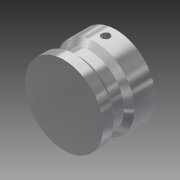
# Autodesk Inventor part: wheel_hub
Saved by Autodesk Inventor 2013 (Build 170138000, 138)
## iProperties
Created: 2013-07-22
Part Number: wheel_hub
Material: Generic
Document SubType Name: Modeling
Designer: dkboone
Density: 1 g/cm^3
Author: dkboone
Autodesk Inventor part; units mm, degrees
note: some values were not read from the file. Chosen so that the rebuilt part matches the saved one: direction of "Hole2".
ref_plane "YZ Plane" through (0, 0, 0) normal (1, 0, 0) x (0, 1, 0)
ref_plane "XY Plane" through (0, 0, 0) normal (0, 0, 1) x (1, 0, 0)
sketch "Sketch1" plane through (0, 0, 0) normal (1, 0, 0) x (0, 1, 0)
  line L0 (0, 0) -> (9.525, 0)
  line L1 (9.525, 0) -> (9.525, -2.54)
  line L2 (9.525, -2.54) -> (8.255, -3.81)
  line L3 (8.255, -3.81) -> (8.255, -6.35)
  line L4 (8.255, -6.35) -> (9.525, -7.62)
  line L5 (9.525, -7.62) -> (9.525, -12.7)
  line L6 (9.525, -12.7) -> (0, -12.7)
  line L7 (0, -12.7) -> (0, 0)
  line L8 (0, -15.24) -> (0, 2.54) projected
  dimension "d0" = 9.525
  dimension "d1" = 135
  dimension "d2" = 2.54
  dimension "d4" = 1.27
  dimension "d5" = 12.7
  dimension "d7" = 2.54
  constraints: 16 end point, 4 perpendicular, 2 collinear, 1 horizontal, 1 parallel
  measures "d0" distance from line of L0.start L1
  measures "d1" angle of L1 L2
  measures "d2" distance of L0.end L1.end
  measures "d4" distance between parallel lines of L3 L5
  measures "d5" distance between parallel lines of L6 L0
  measures "d7" distance of L2.end L3.end
revolve "Revolution1" add sketch "Sketch1" angle 360 about axis through (0, 0, -10) along (0, 0, 1)
sketch "Sketch2" plane through (0, 0, -12.7) normal (0, 0, -1) x (-1, 0, 0)
  circle A0 centre (0, 0) radius 9.525 projected
  constraints: 1 coincident
hole "Hole1" at (0, 0, -12.7) direction (0, 0, 1) diameter 5 depth 11.1125 tip angle 118
ref_plane "Work Plane1" through (0, 9.525, -10.16) normal (0, 1, 0) x (-1, 0, 0)
sketch "Sketch3" plane through (0, 9.525, -10.16) normal (0, 1, 0) x (-1, 0, 0)
  line L0 (0, 10.16) -> (0, 0) construction
  dimension "d16" = 10.16
  constraints: 2 end point, 1 vertical
  measures "d16" distance of L0.end L0.start
hole "Hole2" at (0, 9.525, -10.16) direction (0, -1, 0) diameter 2 end up to surface
body "Solid1"
